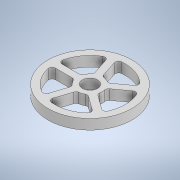
# Autodesk Inventor part: 8_21mm
Saved by Autodesk Inventor 2020 (Build 240168000, 168)
## iProperties
Created: 2021-02-20
Part Number: 8_21mm
Material: Generic
Document SubType Name: Modeling
Designer: Shuang Peng
Density: 1 g/cm^3
Appearance: Default
Author: Shuang Peng
Autodesk Inventor part; units mm, degrees
ref_plane "YZ Plane" through (0, 0, 0) normal (1, 0, 0) x (0, 1, 0)
ref_plane "XZ Plane" through (0, 0, 0) normal (0, 1, 0) x (-1, 0, 0)
ref_plane "XY Plane" through (0, 0, 0) normal (0, 0, 1) x (1, 0, 0)
sketch "Sketch1" plane through (0, 0, 0) normal (0, 1, 0) x (-1, 0, 0)
  circle A0 centre (0, 0) radius 4.5
  circle A1 centre (0, 0) radius 25
  circle A2 centre (0, 0) radius 7.5
  circle A3 centre (0, 0) radius 21
  line L0 (0, 0) -> (25, 0)
  line L1 (22.5, 2) -> (22.5, -2)
  line L2 (22.5, -2) -> (2.5, -2)
  line L3 (2.5, -2) -> (2.5, 2)
  line L4 (2.5, 2) -> (22.5, 2)
  line L5 (22.5, 2) -> (2.5, -2) construction
  line L6 (22.5, -2) -> (2.5, 2) construction
  line L7 (5.0508, 22.0168) -> (8.855, 20.7807)
  line L8 (-1.1296, 2.9957) -> (5.0508, 22.0168)
  line L9 (8.855, 20.7807) -> (2.6747, 1.7596)
  line L10 (2.6747, 1.7596) -> (-1.1296, 2.9957)
  line L11 (-19.3785, 11.6071) -> (-17.0273, 14.8432)
  line L12 (-3.1981, -0.1486) -> (-19.3785, 11.6071)
  line L13 (-17.0273, 14.8432) -> (-0.847, 3.0875)
  line L14 (-0.847, 3.0875) -> (-3.1981, -0.1486)
  line L15 (-17.0273, -14.8432) -> (-19.3785, -11.6071)
  line L16 (-0.847, -3.0875) -> (-17.0273, -14.8432)
  line L17 (-19.3785, -11.6071) -> (-3.1981, 0.1486)
  line L18 (-3.1981, 0.1486) -> (-0.847, -3.0875)
  line L19 (8.855, -20.7807) -> (5.0508, -22.0168)
  line L20 (2.6747, -1.7596) -> (8.855, -20.7807)
  line L21 (5.0508, -22.0168) -> (-1.1296, -2.9957)
  line L22 (-1.1296, -2.9957) -> (2.6747, -1.7596)
  point P0 (12.5, 0)
  point P1 (7.2284, -2)
  point P2 (20.9045, -2)
  point P3 (8.362, -19.2634)
  point P4 (4.1358, -6.2566)
  point P5 (7.2284, 2)
  point P6 (4.1358, 6.2566)
  point P7 (8.362, 19.2634)
  point P8 (20.9045, 2)
  point P9 (0.3316, 7.4927)
  point P10 (-4.6723, 5.8668)
  point P11 (-15.7366, 13.9054)
  point P12 (4.5577, 20.4994)
  point P13 (-4.6723, -5.8668)
  point P14 (0.3316, -7.4927)
  point P15 (4.5577, -20.4994)
  point P16 (-15.7366, -13.9054)
  point P17 (-7.0235, 2.6307)
  point P18 (-7.0235, -2.6307)
  point P19 (-18.0877, -10.6693)
  point P20 (-18.0877, 10.6693)
  dimension "d1" = 50
  dimension "d0" = 9
  dimension "d2" = 3
  dimension "d3" = 4
  dimension "d4" = 4
  dimension "d5" = 20
  dimension "d8" = 360
  constraints: 46 end point, 4 coincident, 3 centre point, 3 midpoint, 2 parallel, 2 perpendicular, 1 horizontal, 1 horizontal alignment, 43 other
  measures "d0" diameter of A0
  measures "d2" radial gap between concentric circles of A2 A0
  measures "d4" distance of L1.start L1.end
  measures "d5" distance of L1.end L2.end
extrude "Extrusion1" add sketch "Sketch1" along normal blind 6 contours L0 A2 L2 A0 | A0 L4 A2 L0 | A0 L9 A2 L4 | L2 A2 L20 A0 | L0 A3 L2 A2 | A2 L4 A3 L0 | A0 L8 A2 L9 | L20 A2 L21 A0 | L0 L1 L2 A3 | A3 L4 L1 L0 | A0 L13 A2 L8 | A2 L8 A3 L9 | L21 A2 L16 A0 | L20 A3 L21 A2 | A0 L12 A2 L13 | A3 L8 L7 L9 | L16 A2 L17 A0 | L20 L19 L21 A3 | A0 L17 A2 L12 | A2 L12 A3 L13 | L16 A3 L17 A2 | A3 L12 L11 L13 | L16 L15 L17 A3 | A1
fillet "Fillet1" radius 2 4 edges at (-8.362, 3, 19.2634) (-20.9045, 3, 2) (-7.2284, 3, 2) (-4.1358, 3, 6.2566)
pattern_circular "Circular Pattern1" count 5 over 360 about axis through (0, 0, 0) along (0, 1, 0) of "Fillet1"
body "Solid1"
